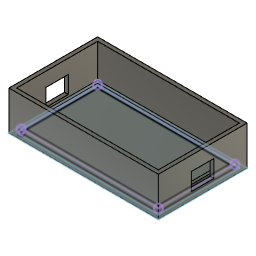
Krabickabezvrsku (Autodesk Fusion 360 design; units mm, degrees)
Autodesk Fusion 360 part; units mm, degrees
sketch "Spodek" plane through (0, 0, 0) normal (0, 0, 1) x (1, 0, 0)
  line L0 (0, 0) -> (61, 0)
  line L1 (61, 0) -> (61, 34)
  line L2 (61, 34) -> (0, 34)
  line L3 (0, 34) -> (0, 0)
  line L4 (-1, 35) -> (62, 35)
  line L5 (62, 35) -> (62, -1)
  line L6 (62, -1) -> (-1, -1)
  line L7 (-1, -1) -> (-1, 35)
  line L8 (-2.7, -2.7) -> (-2.7, 36.7) construction
  line L9 (63.7, 36.7) -> (-2.7, 36.7) construction
  line L10 (63.7, -2.7) -> (63.7, 36.7) construction
  line L11 (63.7, -2.7) -> (-2.7, -2.7) construction
  line L12 (-2.7, -2.7) -> (63.7, -2.7)
  line L13 (63.7, -2.7) -> (63.7, 36.7)
  line L14 (63.7, 36.7) -> (-2.7, 36.7)
  line L15 (-2.7, 36.7) -> (-2.7, -2.7)
  dimension "d1" = 61
  dimension "d2" = 34
  dimension "d3" = 63
  dimension "d4" = 36
  dimension "d5" = 1.7
  dimension "d6" = 1.7
  dimension "d7" = 1.7
  dimension "d8" = 1.7
  constraint horizontal L0
  constraint vertical L1
  constraint horizontal L2
  constraint vertical L3
  constraint coincident L0.start L3.end
  constraint horizontal L4
  constraint vertical L5
  constraint horizontal L6
  constraint vertical L7
  constraint vertical L8
  constraint perpendicular L8 L9
  constraint perpendicular L9 L10
  constraint perpendicular L10 L11
  constraint horizontal L12
  constraint vertical L13
  constraint horizontal L14
  constraint vertical L15
  measures "d1" distance of L0.start L0.end
  measures "d2" distance of L0.start L2.end
  measures "d3" distance of L4.start L4.end
  measures "d4" distance of L4.start L6.end
  measures "d5" distance of L7 L8
  measures "d6" distance of L4 L9
  measures "d7" distance of L5 L10
  measures "d8" distance of L6 L11
sketch "TotoNevim" plane through (0, 0, 0) normal (0, 0, 1) x (1, 0, 0)
extrude "Extrude1" add sketch "Spodek" along normal blind 12 contours L12 L13 L14 L15
extrude "Extrude2" add sketch "Spodek" along normal blind 1.5 contours L0 L1 L2 L3 | L4 L5 L6 L7
sketch "Sketch3" plane through (0, 0, 1.5) normal (0, 0, 1) x (-1, 0, 0)
  line L0 (1, 1) -> (-62, 1)
  line L1 (-62, 1) -> (-62, -35)
  line L2 (-62, -35) -> (1, -35)
  line L3 (1, -35) -> (1, 1)
  line L4 (-59.78, -32.78) -> (-1.22, -32.78)
  line L5 (-1.22, -32.78) -> (-1.22, -1.22)
  line L6 (-1.22, -1.22) -> (-59.78, -1.22)
  line L7 (-59.78, -1.22) -> (-59.78, -32.78)
  line L8 (-61, 0) -> (-61, -34)
  line L9 (0, 0) -> (-61, 0)
  line L10 (0, -34) -> (0, 0)
  line L11 (-61, -34) -> (0, -34)
  dimension "d13" = 1.22
  dimension "d14" = 1.22
  dimension "d15" = 1.22
  dimension "d16" = 1.22
  constraint horizontal L4
  constraint vertical L5
  constraint horizontal L6
  constraint vertical L7
  measures "d13" distance of L7 L8
  measures "d14" distance of L6 L9
  measures "d15" distance of L5 L10
  measures "d16" distance of L4 L11
extrude "Extrude3" add sketch "Sketch3" along normal blind 1.8 contours L8 L9 L10 L11
extrude "Extrude4" add 1 faces at (20, -2.1333, 12) along direction (0, 0, 1) blind 5.243
extrude "Extrude5" add 1 faces at (20, -2.1333, 17.243) along direction (0, 0, 1) blind 0.021
sketch "Prurez1" plane through (-2.7, 0, 0) normal (-1, 0, 0) x (0, -1, 0)
  line L0 (-36.7, 0) -> (2.7, 0)
  line L1 (2.7, 0) -> (2.7, 17.264)
  line L2 (2.7, 17.264) -> (-36.7, 17.264)
  line L3 (-36.7, 17.264) -> (-36.7, 0)
  line L4 (-12, 3.3) -> (-12, 11) construction
  line L5 (0, 1.5) -> (0, 3.3) construction
  line L6 (-22, 11) -> (-22, 3.3) construction
  line L7 (-34, 3.3) -> (-34, 11) construction
  line L8 (-35, 1.5) -> (-35, 17.264) construction
  line L9 (-22, 11) -> (-12, 11) construction
  line L10 (-12, 11) -> (-12, 3.3) construction
  line L11 (-12, 3.3) -> (-22, 3.3) construction
  line L12 (-22, 3.3) -> (-22, 11) construction
  line L13 (-22, 11) -> (-12, 11)
  line L14 (-12, 11) -> (-12, 3.3)
  line L15 (-12, 3.3) -> (-22, 3.3)
  line L16 (-22, 3.3) -> (-22, 11)
  dimension "d23" = 7.7
  dimension "d24" = 12
  dimension "d25" = 12
  dimension "d26" = 1
  constraint perpendicular L2 L4
  constraint parallel L4 L6
  constraint perpendicular L2 L7
  constraint horizontal L9
  constraint vertical L10
  constraint horizontal L11
  constraint vertical L12
  constraint horizontal L13
  constraint vertical L14
  constraint horizontal L15
  constraint vertical L16
  measures "d23" distance of L4.start L4.end
  measures "d24" distance of L4 L5
  measures "d25" distance of L6 L7
  measures "d26" distance of L7 L8
extrude "Extrude6" cut sketch "Prurez1" against normal up to surface (66.4 mm away) contours L13 L14 L15 L16
equation "d19 = 14 mm - 8.757 mm"
equation "d21 = 14 mm - 13.979 mm"
